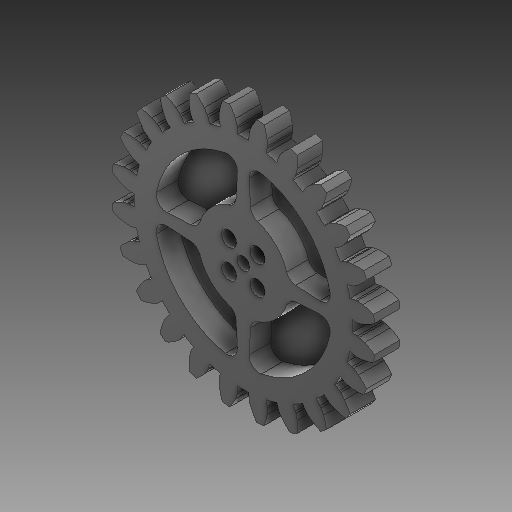
# Autodesk Inventor part: 歯車m2.z24
Saved by Autodesk Inventor 2020 (Build 240168000, 168)
## iProperties
Created: 2019-09-03
Part Number: 歯車m2.z24
Material: アセタール樹脂、黒
Document SubType Name: Modeling
Designer: 雪村
Density: 1.425 g/cm^3
Appearance: 滑らか - 黒
Mass: 8.68564 g
Surface Area: 61.5499 cm^2
Volume: 6.09519 cm^3
Description: ジュラコン 5t
Author: 雪村
Autodesk Inventor part; units mm, degrees
ref_plane "YZ Plane" through (0, 0, 0) normal (1, 0, 0) x (0, 1, 0)
ref_plane "XZ Plane" through (0, 0, 0) normal (0, 1, 0) x (-1, 0, 0)
ref_plane "XY Plane" through (0, 0, 0) normal (0, 0, 1) x (1, 0, 0)
sketch "スケッチ1" plane through (0, 0, 0) normal (0, 0, 1) x (1, 0, 0)
  arc A0 (1.1972, 22.8655) -> (1.1394, 22.5238) centre (3.3501, 22.3258) ccw
  arc A1 (1.5628, 23.9329) -> (1.1972, 22.8655) centre (7.1312, 21.4295) ccw
  arc A2 (2.6831, 25.8612) -> (1.5628, 23.9329) centre (11.2055, 19.6203) ccw
  arc A3 (-4.7616, 22.3962) -> (-4.729, 22.0512) centre (-2.5424, 22.4322) ccw
  arc A4 (-4.6848, 23.5219) -> (-4.7616, 22.3962) centre (1.3418, 22.545) ccw
  arc A5 (-4.1017, 25.6744) -> (-4.6848, 23.5219) centre (5.7456, 21.852) ccw
  arc A6 (-10.3959, 20.4007) -> (-10.2751, 20.0759) centre (-8.2616, 21.0098) ccw
  arc A7 (-10.613, 21.5079) -> (-10.3959, 20.4007) centre (-4.539, 22.1241) ccw
  arc A8 (-10.607, 23.738) -> (-10.613, 21.5079) centre (-0.1059, 22.5945) ccw
  arc A9 (-15.3218, 17.0149) -> (-15.121, 16.7325) centre (-13.4178, 18.1556) ccw
  arc A10 (-15.8181, 18.0282) -> (-15.3218, 17.0149) centre (-10.1104, 20.1955) ccw
  arc A11 (-16.3894, 20.1838) -> (-15.8181, 18.0282) centre (-5.9502, 21.7972) ccw
  arc A12 (-19.2035, 12.4696) -> (-18.9365, 12.2487) centre (-17.6597, 14.0642) ccw
  arc A13 (-19.9451, 13.3199) -> (-19.2035, 12.4696) centre (-14.9929, 16.8905) ccw
  arc A14 (-21.0549, 15.2542) -> (-19.9451, 13.3199) centre (-11.389, 19.5144) ccw
  arc A15 (-21.7765, 7.0744) -> (-21.4614, 6.9302) centre (-20.698, 9.0143) ccw
  arc A16 (-22.713, 7.7038) -> (-21.7765, 7.0744) centre (-18.8536, 12.4346) ccw
  arc A17 (-24.2856, 9.285) -> (-22.713, 7.7038) centre (-16.0516, 15.9018) ccw
  arc A18 (-22.8655, 1.1972) -> (-22.5238, 1.1394) centre (-22.3258, 3.3501) ccw
  arc A19 (-23.9329, 1.5628) -> (-22.8655, 1.1972) centre (-21.4295, 7.1312) ccw
  arc A20 (-25.8612, 2.6831) -> (-23.9329, 1.5628) centre (-19.6203, 11.2055) ccw
  arc A21 (-22.3962, -4.7616) -> (-22.0512, -4.729) centre (-22.4322, -2.5424) ccw
  arc A22 (-23.5219, -4.6848) -> (-22.3962, -4.7616) centre (-22.545, 1.3418) ccw
  arc A23 (-25.6744, -4.1017) -> (-23.5219, -4.6848) centre (-21.852, 5.7456) ccw
  arc A24 (-20.4007, -10.3959) -> (-20.0759, -10.2751) centre (-21.0098, -8.2616) ccw
  arc A25 (-21.5079, -10.613) -> (-20.4007, -10.3959) centre (-22.1241, -4.539) ccw
  arc A26 (-23.738, -10.607) -> (-21.5079, -10.613) centre (-22.5945, -0.1059) ccw
  arc A27 (-17.0149, -15.3218) -> (-16.7325, -15.121) centre (-18.1556, -13.4178) ccw
  arc A28 (-18.0282, -15.8181) -> (-17.0149, -15.3218) centre (-20.1955, -10.1104) ccw
  arc A29 (-20.1838, -16.3894) -> (-18.0282, -15.8181) centre (-21.7972, -5.9502) ccw
  arc A30 (-12.4696, -19.2035) -> (-12.2487, -18.9365) centre (-14.0642, -17.6597) ccw
  arc A31 (-13.3199, -19.9451) -> (-12.4696, -19.2035) centre (-16.8905, -14.9929) ccw
  arc A32 (-15.2542, -21.0549) -> (-13.3199, -19.9451) centre (-19.5144, -11.389) ccw
  arc A33 (-7.0744, -21.7765) -> (-6.9302, -21.4614) centre (-9.0143, -20.698) ccw
  arc A34 (-7.7038, -22.713) -> (-7.0744, -21.7765) centre (-12.4346, -18.8536) ccw
  arc A35 (-9.285, -24.2856) -> (-7.7038, -22.713) centre (-15.9018, -16.0516) ccw
  arc A36 (-1.1972, -22.8655) -> (-1.1394, -22.5238) centre (-3.3501, -22.3258) ccw
  arc A37 (-1.5628, -23.9329) -> (-1.1972, -22.8655) centre (-7.1312, -21.4295) ccw
  arc A38 (-2.6831, -25.8612) -> (-1.5628, -23.9329) centre (-11.2055, -19.6203) ccw
  arc A39 (4.7616, -22.3962) -> (4.729, -22.0512) centre (2.5424, -22.4322) ccw
  arc A40 (4.6848, -23.5219) -> (4.7616, -22.3962) centre (-1.3418, -22.545) ccw
  arc A41 (4.1017, -25.6744) -> (4.6848, -23.5219) centre (-5.7456, -21.852) ccw
  arc A42 (10.3959, -20.4007) -> (10.2751, -20.0759) centre (8.2616, -21.0098) ccw
  arc A43 (10.613, -21.5079) -> (10.3959, -20.4007) centre (4.539, -22.1241) ccw
  arc A44 (10.607, -23.738) -> (10.613, -21.5079) centre (0.1059, -22.5945) ccw
  arc A45 (15.3218, -17.0149) -> (15.121, -16.7325) centre (13.4178, -18.1556) ccw
  arc A46 (15.8181, -18.0282) -> (15.3218, -17.0149) centre (10.1104, -20.1955) ccw
  arc A47 (16.3894, -20.1838) -> (15.8181, -18.0282) centre (5.9502, -21.7972) ccw
  arc A48 (19.2035, -12.4696) -> (18.9365, -12.2487) centre (17.6597, -14.0642) ccw
  arc A49 (19.9451, -13.3199) -> (19.2035, -12.4696) centre (14.9929, -16.8905) ccw
  arc A50 (21.0549, -15.2542) -> (19.9451, -13.3199) centre (11.389, -19.5144) ccw
  arc A51 (21.7765, -7.0744) -> (21.4614, -6.9302) centre (20.698, -9.0143) ccw
  arc A52 (22.713, -7.7038) -> (21.7765, -7.0744) centre (18.8536, -12.4346) ccw
  arc A53 (24.2856, -9.285) -> (22.713, -7.7038) centre (16.0516, -15.9018) ccw
  arc A54 (22.8655, -1.1972) -> (22.5238, -1.1394) centre (22.3258, -3.3501) ccw
  arc A55 (23.9329, -1.5628) -> (22.8655, -1.1972) centre (21.4295, -7.1312) ccw
  arc A56 (25.8612, -2.6831) -> (23.9329, -1.5628) centre (19.6203, -11.2055) ccw
  arc A57 (22.3962, 4.7616) -> (22.0512, 4.729) centre (22.4322, 2.5424) ccw
  arc A58 (23.5219, 4.6848) -> (22.3962, 4.7616) centre (22.545, -1.3418) ccw
  arc A59 (25.6744, 4.1017) -> (23.5219, 4.6848) centre (21.852, -5.7456) ccw
  arc A60 (20.4007, 10.3959) -> (20.0759, 10.2751) centre (21.0098, 8.2616) ccw
  arc A61 (21.5079, 10.613) -> (20.4007, 10.3959) centre (22.1241, 4.539) ccw
  arc A62 (23.738, 10.607) -> (21.5079, 10.613) centre (22.5945, 0.1059) ccw
  arc A63 (17.0149, 15.3218) -> (16.7325, 15.121) centre (18.1556, 13.4178) ccw
  arc A64 (18.0282, 15.8181) -> (17.0149, 15.3218) centre (20.1955, 10.1104) ccw
  arc A65 (20.1838, 16.3894) -> (18.0282, 15.8181) centre (21.7972, 5.9502) ccw
  arc A66 (12.4696, 19.2035) -> (12.2487, 18.9365) centre (14.0642, 17.6597) ccw
  arc A67 (13.3199, 19.9451) -> (12.4696, 19.2035) centre (16.8905, 14.9929) ccw
  arc A68 (15.2542, 21.0549) -> (13.3199, 19.9451) centre (19.5144, 11.389) ccw
  arc A69 (7.0744, 21.7765) -> (6.9302, 21.4614) centre (9.0143, 20.698) ccw
  arc A70 (7.7038, 22.713) -> (7.0744, 21.7765) centre (12.4346, 18.8536) ccw
  arc A71 (9.285, 24.2856) -> (7.7038, 22.713) centre (15.9018, 16.0516) ccw
  arc A72 (-1.1394, 22.5238) -> (-1.1972, 22.8655) centre (-3.3501, 22.3258) ccw
  arc A73 (-1.1972, 22.8655) -> (-1.5628, 23.9329) centre (-7.1312, 21.4295) ccw
  arc A74 (-1.5628, 23.9329) -> (-2.6831, 25.8612) centre (-11.2055, 19.6203) ccw
  arc A75 (-6.9302, 21.4614) -> (-7.0744, 21.7765) centre (-9.0143, 20.698) ccw
  arc A76 (-7.0744, 21.7765) -> (-7.7038, 22.713) centre (-12.4346, 18.8536) ccw
  arc A77 (-7.7038, 22.713) -> (-9.285, 24.2856) centre (-15.9018, 16.0516) ccw
  arc A78 (-12.2487, 18.9365) -> (-12.4696, 19.2035) centre (-14.0642, 17.6597) ccw
  arc A79 (-12.4696, 19.2035) -> (-13.3199, 19.9451) centre (-16.8905, 14.9929) ccw
  arc A80 (-13.3199, 19.9451) -> (-15.2542, 21.0549) centre (-19.5144, 11.389) ccw
  arc A81 (-16.7325, 15.121) -> (-17.0149, 15.3218) centre (-18.1556, 13.4178) ccw
  arc A82 (-17.0149, 15.3218) -> (-18.0282, 15.8181) centre (-20.1955, 10.1104) ccw
  arc A83 (-18.0282, 15.8181) -> (-20.1838, 16.3894) centre (-21.7972, 5.9502) ccw
  arc A84 (-20.0759, 10.2751) -> (-20.4007, 10.3959) centre (-21.0098, 8.2616) ccw
  arc A85 (-20.4007, 10.3959) -> (-21.5079, 10.613) centre (-22.1241, 4.539) ccw
  arc A86 (-21.5079, 10.613) -> (-23.738, 10.607) centre (-22.5945, 0.1059) ccw
  arc A87 (-22.0512, 4.729) -> (-22.3962, 4.7616) centre (-22.4322, 2.5424) ccw
  arc A88 (-22.3962, 4.7616) -> (-23.5219, 4.6848) centre (-22.545, -1.3418) ccw
  arc A89 (-23.5219, 4.6848) -> (-25.6744, 4.1017) centre (-21.852, -5.7456) ccw
  arc A90 (-22.5238, -1.1394) -> (-22.8655, -1.1972) centre (-22.3258, -3.3501) ccw
  arc A91 (-22.8655, -1.1972) -> (-23.9329, -1.5628) centre (-21.4295, -7.1312) ccw
  arc A92 (-23.9329, -1.5628) -> (-25.8612, -2.6831) centre (-19.6203, -11.2055) ccw
  arc A93 (-21.4614, -6.9302) -> (-21.7765, -7.0744) centre (-20.698, -9.0143) ccw
  arc A94 (-21.7765, -7.0744) -> (-22.713, -7.7038) centre (-18.8536, -12.4346) ccw
  arc A95 (-22.713, -7.7038) -> (-24.2856, -9.285) centre (-16.0516, -15.9018) ccw
  arc A96 (-18.9365, -12.2487) -> (-19.2035, -12.4696) centre (-17.6597, -14.0642) ccw
  arc A97 (-19.2035, -12.4696) -> (-19.9451, -13.3199) centre (-14.9929, -16.8905) ccw
  arc A98 (-19.9451, -13.3199) -> (-21.0549, -15.2542) centre (-11.389, -19.5144) ccw
  arc A99 (-15.121, -16.7325) -> (-15.3218, -17.0149) centre (-13.4178, -18.1556) ccw
  arc A100 (-15.3218, -17.0149) -> (-15.8181, -18.0282) centre (-10.1104, -20.1955) ccw
  arc A101 (-15.8181, -18.0282) -> (-16.3894, -20.1838) centre (-5.9502, -21.7972) ccw
  arc A102 (-10.2751, -20.0759) -> (-10.3959, -20.4007) centre (-8.2616, -21.0098) ccw
  arc A103 (-10.3959, -20.4007) -> (-10.613, -21.5079) centre (-4.539, -22.1241) ccw
  arc A104 (-10.613, -21.5079) -> (-10.607, -23.738) centre (-0.1059, -22.5945) ccw
  arc A105 (-4.729, -22.0512) -> (-4.7616, -22.3962) centre (-2.5424, -22.4322) ccw
  arc A106 (-4.7616, -22.3962) -> (-4.6848, -23.5219) centre (1.3418, -22.545) ccw
  arc A107 (-4.6848, -23.5219) -> (-4.1017, -25.6744) centre (5.7456, -21.852) ccw
  arc A108 (1.1394, -22.5238) -> (1.1972, -22.8655) centre (3.3501, -22.3258) ccw
  arc A109 (1.1972, -22.8655) -> (1.5628, -23.9329) centre (7.1312, -21.4295) ccw
  arc A110 (1.5628, -23.9329) -> (2.6831, -25.8612) centre (11.2055, -19.6203) ccw
  arc A111 (6.9302, -21.4614) -> (7.0744, -21.7765) centre (9.0143, -20.698) ccw
  arc A112 (7.0744, -21.7765) -> (7.7038, -22.713) centre (12.4346, -18.8536) ccw
  arc A113 (7.7038, -22.713) -> (9.285, -24.2856) centre (15.9018, -16.0516) ccw
  arc A114 (12.2487, -18.9365) -> (12.4696, -19.2035) centre (14.0642, -17.6597) ccw
  arc A115 (12.4696, -19.2035) -> (13.3199, -19.9451) centre (16.8905, -14.9929) ccw
  arc A116 (13.3199, -19.9451) -> (15.2542, -21.0549) centre (19.5144, -11.389) ccw
  arc A117 (16.7325, -15.121) -> (17.0149, -15.3218) centre (18.1556, -13.4178) ccw
  arc A118 (17.0149, -15.3218) -> (18.0282, -15.8181) centre (20.1955, -10.1104) ccw
  arc A119 (18.0282, -15.8181) -> (20.1838, -16.3894) centre (21.7972, -5.9502) ccw
  arc A120 (20.0759, -10.2751) -> (20.4007, -10.3959) centre (21.0098, -8.2616) ccw
  arc A121 (20.4007, -10.3959) -> (21.5079, -10.613) centre (22.1241, -4.539) ccw
  arc A122 (21.5079, -10.613) -> (23.738, -10.607) centre (22.5945, -0.1059) ccw
  arc A123 (22.0512, -4.729) -> (22.3962, -4.7616) centre (22.4322, -2.5424) ccw
  arc A124 (22.3962, -4.7616) -> (23.5219, -4.6848) centre (22.545, 1.3418) ccw
  arc A125 (23.5219, -4.6848) -> (25.6744, -4.1017) centre (21.852, 5.7456) ccw
  arc A126 (22.5238, 1.1394) -> (22.8655, 1.1972) centre (22.3258, 3.3501) ccw
  arc A127 (22.8655, 1.1972) -> (23.9329, 1.5628) centre (21.4295, 7.1312) ccw
  arc A128 (23.9329, 1.5628) -> (25.8612, 2.6831) centre (19.6203, 11.2055) ccw
  arc A129 (21.4614, 6.9302) -> (21.7765, 7.0744) centre (20.698, 9.0143) ccw
  arc A130 (21.7765, 7.0744) -> (22.713, 7.7038) centre (18.8536, 12.4346) ccw
  arc A131 (22.713, 7.7038) -> (24.2856, 9.285) centre (16.0516, 15.9018) ccw
  arc A132 (18.9365, 12.2487) -> (19.2035, 12.4696) centre (17.6597, 14.0642) ccw
  arc A133 (19.2035, 12.4696) -> (19.9451, 13.3199) centre (14.9929, 16.8905) ccw
  arc A134 (19.9451, 13.3199) -> (21.0549, 15.2542) centre (11.389, 19.5144) ccw
  arc A135 (15.121, 16.7325) -> (15.3218, 17.0149) centre (13.4178, 18.1556) ccw
  arc A136 (15.3218, 17.0149) -> (15.8181, 18.0282) centre (10.1104, 20.1955) ccw
  arc A137 (15.8181, 18.0282) -> (16.3894, 20.1838) centre (5.9502, 21.7972) ccw
  arc A138 (10.2751, 20.0759) -> (10.3959, 20.4007) centre (8.2616, 21.0098) ccw
  arc A139 (10.3959, 20.4007) -> (10.613, 21.5079) centre (4.539, 22.1241) ccw
  arc A140 (10.613, 21.5079) -> (10.607, 23.738) centre (0.1059, 22.5945) ccw
  arc A141 (4.729, 22.0512) -> (4.7616, 22.3962) centre (2.5424, 22.4322) ccw
  arc A142 (4.7616, 22.3962) -> (4.6848, 23.5219) centre (-1.3418, 22.545) ccw
  arc A143 (4.6848, 23.5219) -> (4.1017, 25.6744) centre (-5.7456, 21.852) ccw
  arc A144 (1.0863, 21.4725) -> (-1.0863, 21.4725) centre (0, 0) ccw
  arc A145 (-4.5083, 21.022) -> (-6.6068, 20.4597) centre (0, 0) ccw
  arc A146 (-9.7955, 19.1389) -> (-11.677, 18.0526) centre (0, 0) ccw
  arc A147 (-14.4153, 15.9515) -> (-15.9515, 14.4153) centre (0, 0) ccw
  arc A148 (-18.0526, 11.677) -> (-19.1389, 9.7955) centre (0, 0) ccw
  arc A149 (-20.4597, 6.6068) -> (-21.022, 4.5083) centre (0, 0) ccw
  arc A150 (-21.4725, 1.0863) -> (-21.4725, -1.0863) centre (0, 0) ccw
  arc A151 (-21.022, -4.5083) -> (-20.4597, -6.6068) centre (0, 0) ccw
  arc A152 (-19.1389, -9.7955) -> (-18.0526, -11.677) centre (0, 0) ccw
  arc A153 (-15.9515, -14.4153) -> (-14.4153, -15.9515) centre (0, 0) ccw
  arc A154 (-11.677, -18.0526) -> (-9.7955, -19.1389) centre (0, 0) ccw
  arc A155 (-6.6068, -20.4597) -> (-4.5083, -21.022) centre (0, 0) ccw
  arc A156 (-1.0863, -21.4725) -> (1.0863, -21.4725) centre (0, 0) ccw
  arc A157 (4.5083, -21.022) -> (6.6068, -20.4597) centre (0, 0) ccw
  arc A158 (9.7955, -19.1389) -> (11.677, -18.0526) centre (0, 0) ccw
  arc A159 (14.4153, -15.9515) -> (15.9515, -14.4153) centre (0, 0) ccw
  arc A160 (18.0526, -11.677) -> (19.1389, -9.7955) centre (0, 0) ccw
  arc A161 (20.4597, -6.6068) -> (21.022, -4.5083) centre (0, 0) ccw
  arc A162 (21.4725, -1.0863) -> (21.4725, 1.0863) centre (0, 0) ccw
  arc A163 (21.022, 4.5083) -> (20.4597, 6.6068) centre (0, 0) ccw
  arc A164 (19.1389, 9.7955) -> (18.0526, 11.677) centre (0, 0) ccw
  arc A165 (15.9515, 14.4153) -> (14.4153, 15.9515) centre (0, 0) ccw
  arc A166 (11.677, 18.0526) -> (9.7955, 19.1389) centre (0, 0) ccw
  arc A167 (6.6068, 20.4597) -> (4.5083, 21.022) centre (0, 0) ccw
  arc A168 (-2.6831, 25.8612) -> (-4.1017, 25.6744) centre (0, 0) ccw
  arc A169 (-9.285, 24.2856) -> (-10.607, 23.738) centre (0, 0) ccw
  arc A170 (-15.2542, 21.0549) -> (-16.3894, 20.1838) centre (0, 0) ccw
  arc A171 (-20.1838, 16.3894) -> (-21.0549, 15.2542) centre (0, 0) ccw
  arc A172 (-23.738, 10.607) -> (-24.2856, 9.285) centre (0, 0) ccw
  arc A173 (-25.6744, 4.1017) -> (-25.8612, 2.6831) centre (0, 0) ccw
  arc A174 (-25.8612, -2.6831) -> (-25.6744, -4.1017) centre (0, 0) ccw
  arc A175 (-24.2856, -9.285) -> (-23.738, -10.607) centre (0, 0) ccw
  arc A176 (-21.0549, -15.2542) -> (-20.1838, -16.3894) centre (0, 0) ccw
  arc A177 (-16.3894, -20.1838) -> (-15.2542, -21.0549) centre (0, 0) ccw
  arc A178 (-10.607, -23.738) -> (-9.285, -24.2856) centre (0, 0) ccw
  arc A179 (-4.1017, -25.6744) -> (-2.6831, -25.8612) centre (0, 0) ccw
  arc A180 (2.6831, -25.8612) -> (4.1017, -25.6744) centre (0, 0) ccw
  arc A181 (9.285, -24.2856) -> (10.607, -23.738) centre (0, 0) ccw
  arc A182 (15.2542, -21.0549) -> (16.3894, -20.1838) centre (0, 0) ccw
  arc A183 (20.1838, -16.3894) -> (21.0549, -15.2542) centre (0, 0) ccw
  arc A184 (23.738, -10.607) -> (24.2856, -9.285) centre (0, 0) ccw
  arc A185 (25.6744, -4.1017) -> (25.8612, -2.6831) centre (0, 0) ccw
  arc A186 (25.8612, 2.6831) -> (25.6744, 4.1017) centre (0, 0) ccw
  arc A187 (24.2856, 9.285) -> (23.738, 10.607) centre (0, 0) ccw
  arc A188 (21.0549, 15.2542) -> (20.1838, 16.3894) centre (0, 0) ccw
  arc A189 (16.3894, 20.1838) -> (15.2542, 21.0549) centre (0, 0) ccw
  arc A190 (10.607, 23.738) -> (9.285, 24.2856) centre (0, 0) ccw
  arc A191 (4.1017, 25.6744) -> (2.6831, 25.8612) centre (0, 0) ccw
  line L0 (1.0863, 21.4725) -> (1.1394, 22.5238)
  line L1 (-4.5083, 21.022) -> (-4.729, 22.0512)
  line L2 (-9.7955, 19.1389) -> (-10.2751, 20.0759)
  line L3 (-14.4153, 15.9515) -> (-15.121, 16.7325)
  line L4 (-18.0526, 11.677) -> (-18.9365, 12.2487)
  line L5 (-20.4597, 6.6068) -> (-21.4614, 6.9302)
  line L6 (-21.4725, 1.0863) -> (-22.5238, 1.1394)
  line L7 (-21.022, -4.5083) -> (-22.0512, -4.729)
  line L8 (-19.1389, -9.7955) -> (-20.0759, -10.2751)
  line L9 (-15.9515, -14.4153) -> (-16.7325, -15.121)
  line L10 (-11.677, -18.0526) -> (-12.2487, -18.9365)
  line L11 (-6.6068, -20.4597) -> (-6.9302, -21.4614)
  line L12 (-1.0863, -21.4725) -> (-1.1394, -22.5238)
  line L13 (4.5083, -21.022) -> (4.729, -22.0512)
  line L14 (9.7955, -19.1389) -> (10.2751, -20.0759)
  line L15 (14.4153, -15.9515) -> (15.121, -16.7325)
  line L16 (18.0526, -11.677) -> (18.9365, -12.2487)
  line L17 (20.4597, -6.6068) -> (21.4614, -6.9302)
  line L18 (21.4725, -1.0863) -> (22.5238, -1.1394)
  line L19 (21.022, 4.5083) -> (22.0512, 4.729)
  line L20 (19.1389, 9.7955) -> (20.0759, 10.2751)
  line L21 (15.9515, 14.4153) -> (16.7325, 15.121)
  line L22 (11.677, 18.0526) -> (12.2487, 18.9365)
  line L23 (6.6068, 20.4597) -> (6.9302, 21.4614)
  line L24 (-1.0863, 21.4725) -> (-1.1394, 22.5238)
  line L25 (-6.6068, 20.4597) -> (-6.9302, 21.4614)
  line L26 (-11.677, 18.0526) -> (-12.2487, 18.9365)
  line L27 (-15.9515, 14.4153) -> (-16.7325, 15.121)
  line L28 (-19.1389, 9.7955) -> (-20.0759, 10.2751)
  line L29 (-21.022, 4.5083) -> (-22.0512, 4.729)
  line L30 (-21.4725, -1.0863) -> (-22.5238, -1.1394)
  line L31 (-20.4597, -6.6068) -> (-21.4614, -6.9302)
  line L32 (-18.0526, -11.677) -> (-18.9365, -12.2487)
  line L33 (-14.4153, -15.9515) -> (-15.121, -16.7325)
  line L34 (-9.7955, -19.1389) -> (-10.2751, -20.0759)
  line L35 (-4.5083, -21.022) -> (-4.729, -22.0512)
  line L36 (1.0863, -21.4725) -> (1.1394, -22.5238)
  line L37 (6.6068, -20.4597) -> (6.9302, -21.4614)
  line L38 (11.677, -18.0526) -> (12.2487, -18.9365)
  line L39 (15.9515, -14.4153) -> (16.7325, -15.121)
  line L40 (19.1389, -9.7955) -> (20.0759, -10.2751)
  line L41 (21.022, -4.5083) -> (22.0512, -4.729)
  line L42 (21.4725, 1.0863) -> (22.5238, 1.1394)
  line L43 (20.4597, 6.6068) -> (21.4614, 6.9302)
  line L44 (18.0526, 11.677) -> (18.9365, 12.2487)
  line L45 (14.4153, 15.9515) -> (15.121, 16.7325)
  line L46 (9.7955, 19.1389) -> (10.2751, 20.0759)
  line L47 (4.5083, 21.022) -> (4.729, 22.0512)
  line L48 (-28, 0) -> (28, 0)
  line L49 (0, -28) -> (0, 28)
  line L50 (46, 26) -> (116, 26)
  line L51 (46, 18) -> (116, 18)
  line L52 (46, 10) -> (116, 10)
  line L53 (46, 2) -> (116, 2)
  line L54 (46, -6) -> (116, -6)
  line L55 (46, -14) -> (116, -14)
  line L56 (46, -22) -> (116, -22)
  line L57 (46, -30) -> (116, -30)
  line L58 (46, -38) -> (116, -38)
  line L59 (46, -46) -> (116, -46)
  line L60 (46, -54) -> (116, -54)
  line L61 (46, -62) -> (116, -62)
  line L62 (46, -70) -> (116, -70)
  line L63 (46, 26) -> (46, -70)
  line L64 (116, 26) -> (116, -70)
  line L65 (81, 18) -> (81, -70)
  point P0 (0, 0)
  point P1 (52, 20)
  point P2 (54.5, 12)
  point P3 (54.5, 4)
  point P4 (52, -4)
  point P5 (54.5, -12)
  point P6 (49.5, -20)
  point P7 (52, -28)
  point P8 (52, -36)
  point P9 (52, -44)
  point P10 (54.5, -52)
  point P11 (54.5, -60)
  point P12 (52, -68)
  point P13 (82, 12)
  point P14 (97, 4)
  point P15 (98.25, -4)
  point P16 (94.5, -12)
  point P17 (97, -20)
  point P18 (90.75, -28)
  point P19 (97, -36)
  point P20 (97, -44)
  point P21 (92, -52)
  point P22 (1, 41.5)
  point P23 (1, 35.5)
  point P24 (17.1875, 41.5)
  point P25 (19.3125, 35.5)
  constraints: 288 point on circle, 144 centre point, 128 end point, 14 horizontal, 2 horizontal alignment, 2 midpoint, 2 vertical, 2 vertical alignment, 827 other
extrude "押し出し1" add sketch "スケッチ1" along normal blind 5 contours A1 A2 A191 A143 A142 A141 L47 A167 L23 A69 A70 A71 A190 A140 A139 A138 L46 A166 L22 A66 A67 A68 A189 A137 A136 A135 L45 A165 L21 A63 A64 A65 A188 A134 A133 A132 L44 A164 L20 A60 A61 A62 A187 A131 A130 A129 L43 A163 L19 A57 A58 A59 A186 A128 A127 A126 L42 A162 L48 L49 A144 L0 A0 | L49 L48 A150 L6 A18 A19 A20 A173 A89 A88 A87 L29 A149 L5 A15 A16 A17 A172 A86 A85 A84 L28 A148 L4 A12 A13 A14 A171 A83 A82 A81 L27 A147 L3 A9 A10 A11 A170 A80 A79 A78 L26 A146 L2 A6 A7 A8 A169 A77 A76 A75 L25 A145 L1 A3 A4 A5 A168 A74 A73 A72 L24 A144 | L49 A156 L12 A36 A37 A38 A179 A107 A106 A105 L35 A155 L11 A33 A34 A35 A178 A104 A103 A102 L34 A154 L10 A30 A31 A32 A177 A101 A100 A99 L33 A153 L9 A27 A28 A29 A176 A98 A97 A96 L32 A152 L8 A24 A25 A26 A175 A95 A94 A93 L31 A151 L7 A21 A22 A23 A174 A92 A91 A90 L30 A150 L48 | L48 A162 L18 A54 A55 A56 A185 A125 A124 A123 L41 A161 L17 A51 A52 A53 A184 A122 A121 A120 L40 A160 L16 A48 A49 A50 A183 A119 A118 A117 L39 A159 L15 A45 A46 A47 A182 A116 A115 A114 L38 A158 L14 A42 A43 A44 A181 A113 A112 A111 L37 A157 L13 A39 A40 A41 A180 A110 A109 A108 L36 A156 L49
sketch "スケッチ2" plane through (0, 0, 5) normal (0, 0, 1) x (1, 0, 0)
  line L0 (-2.8, 2.8) -> (2.8, 2.8) construction
  line L1 (2.8, 2.8) -> (2.8, -2.8) construction
  line L2 (2.8, -2.8) -> (-2.8, -2.8) construction
  line L3 (-2.8, -2.8) -> (-2.8, 2.8) construction
  circle A0 centre (-2.8, 2.8) radius 1.5
  circle A1 centre (2.8, 2.8) radius 1.5
  circle A2 centre (2.8, -2.8) radius 1.5
  circle A3 centre (-2.8, -2.8) radius 1.5
  point P0 (0, 0)
  point P1 (0, 0)
  dimension "d2" = 3
  dimension "d3" = 3
  dimension "d4" = 3
  dimension "d5" = 3
  dimension "d6" = 5.6
  constraints: 8 end point, 5 coincident, 4 centre point, 1 horizontal, 9 other
  measures "d2" diameter of A0
  measures "d3" diameter of A1
  measures "d4" diameter of A2
  measures "d5" diameter of A3
  measures "d6" distance of L0.start L0.end
extrude "押し出し2" cut sketch "スケッチ2" against normal through all
sketch "スケッチ3" plane through (0, 0, 5) normal (0, 0, 1) x (1, 0, 0)
  circle A0 centre (0, 0) radius 1.25
  dimension "d9" = 2.5
  constraints: 1 centre point, 1 coincident
  measures "d9" diameter of A0
extrude "押し出し3" cut sketch "スケッチ3" against normal through all
sketch "スケッチ4" plane through (0, 0, 0) normal (0, 0, -1) x (-1, 0, 0)
  circle A0 centre (0, 0) radius 9
  circle A1 centre (0, 0) radius 6
  circle A2 centre (0, 0) radius 17.5
  line L0 (0, 15.6403) -> (0, -15.6403)
  line L1 (-15.4429, 0) -> (15.4429, 0)
  line L2 (-1, 17.4714) -> (-1.5, 8.8741)
  line L3 (1, 17.4714) -> (1.5, 8.8741)
  line L4 (8.8741, 1.5) -> (17.4714, 1)
  line L5 (8.8741, -1.5) -> (17.4714, -1)
  circle A3 centre (0, 0) radius 9
  line L6 (1.5, -8.8741) -> (1, -17.4714)
  line L7 (-17.4714, 1) -> (-8.8741, 1.5)
  line L8 (-17.4714, -1) -> (-8.8741, -1.5)
  line L9 (-1.5, -8.8741) -> (-1, -17.4714)
  circle A4 centre (0, 0) radius 6
  circle A5 centre (0, 0) radius 21.5
  circle A6 centre (0, 0) radius 6
  circle A7 centre (0, 0) radius 1.25 projected
  point P0 (16.9761, 62.7038)
  point P1 (20.9761, 62.7038)
  point P2 (11.2302, 68.4498)
  point P3 (11.2302, 72.4498)
  point P4 (16.9761, 62.7038)
  point P5 (20.9761, 62.7038)
  point P6 (11.2302, 68.4498)
  point P7 (11.2302, 72.4498)
  point P8 (-9.7955, 19.1389)
  point P9 (-2, -7.746)
  point P10 (2, -7.746)
  point P11 (-7.746, -2)
  point P12 (-7.746, 2)
  point P13 (-9.7955, 19.1389)
  point P14 (-1.5, -7.8581)
  point P15 (-7.8581, -1.5)
  point P16 (1.5, -7.8581)
  point P17 (-7.8581, 1.5)
  point P18 (-9.7955, 19.1389)
  dimension "d28" = 4
  dimension "d12" = 1
  dimension "d13" = 1
  dimension "d14" = 1
  dimension "d15" = 1
  dimension "d16" = 1
  dimension "d17" = 1
  dimension "d18" = 1
  dimension "d19" = 1
  dimension "d20" = 1.5
  dimension "d21" = 1.5
  dimension "d22" = 1.5
  dimension "d23" = 1.5
  dimension "d24" = 1.5
  dimension "d25" = 1.5
  dimension "d26" = 1.5
  dimension "d27" = 1.5
  dimension "d29" = 3
  dimension "d30" = 12
  constraints: 20 end point, 5 concentric, 4 centre point, 4 coincident, 4 point on circle, 2 midpoint, 1 horizontal, 1 vertical, 23 other
  measures "d12" distance from line of L0 L2.start
  measures "d13" distance from line of L3.start L0
  measures "d14" distance from line of L1 L4.end
  measures "d15" distance from line of L5.end L1
  measures "d16" distance from line of L0 L6.end
  measures "d17" distance from line of L0 L9.end
  measures "d18" distance from line of L1 L8.start
  measures "d19" distance from line of L1 L7.start
  measures "d20" distance from line of L0 L2.end
  measures "d21" distance from line of L0 L3.end
  measures "d22" distance from line of L1 L4.start
  measures "d23" distance from line of L5.start L1
  measures "d24" distance from line of L0 L6.start
  measures "d25" distance from line of L9.start L0
  measures "d26" distance from line of L1 L8.end
  measures "d27" distance from line of L1 L7.end
  measures "d29" radial gap between concentric circles of A0 A1
  measures "d30" diameter of A1
extrude "押し出し4" cut sketch "スケッチ4" against normal through all contours A0 L3 A2 L4 | L5 A2 L6 A0 | A0 L7 A2 L2 | L9 A2 L8 A0
fillet "フィレット1" radius 2 16 edges at (17.4714, -1, 2.5) (17.4714, 1, 2.5) (8.8741, -1.5, 2.5) (8.8741, 1.5, 2.5) (1.5, 8.8741, 2.5) (-1.5, 8.8741, 2.5) (1, 17.4714, 2.5) (-1, 17.4714, 2.5) (-17.4714, 1, 2.5) (-17.4714, -1, 2.5) (-8.8741, 1.5, 2.5) (-8.8741, -1.5, 2.5) (1.5, -8.8741, 2.5) (-1.5, -8.8741, 2.5) (1, -17.4714, 2.5) (-1, -17.4714, 2.5)
sketch "スケッチ5" plane through (0, 0, 0) normal (0, 0, -1) x (-1, 0, 0)
  arc A0 (-8.5563, -2.791) -> (-2.791, -8.5563) centre (0, 0) ccw projected
  arc A1 (-1.4147, -10.3416) -> (-2.791, -8.5563) centre (-3.4113, -10.4577) ccw projected
  line L0 (-1.4147, -10.3416) -> (-1.1401, -15.0632) projected
  arc A2 (-3.5414, -17.1379) -> (-1.1401, -15.0632) centre (-3.1367, -15.1793) ccw projected
  arc A3 (-17.1379, -3.5414) -> (-3.5414, -17.1379) centre (0, 0) ccw projected
  arc A4 (-15.0632, -1.1401) -> (-17.1379, -3.5414) centre (-15.1793, -3.1367) ccw projected
  line L1 (-15.0632, -1.1401) -> (-10.3416, -1.4147) projected
  arc A5 (-8.5563, -2.791) -> (-10.3416, -1.4147) centre (-10.4577, -3.4113) ccw projected
  line L2 (-1.1401, 15.0632) -> (-1.4147, 10.3416) projected
  arc A6 (-2.791, 8.5563) -> (-1.4147, 10.3416) centre (-3.4113, 10.4577) ccw projected
  arc A7 (-2.791, 8.5563) -> (-8.5563, 2.791) centre (0, 0) ccw projected
  arc A8 (-10.3416, 1.4147) -> (-8.5563, 2.791) centre (-10.4577, 3.4113) ccw projected
  line L3 (-10.3416, 1.4147) -> (-15.0632, 1.1401) projected
  arc A9 (-17.1379, 3.5414) -> (-15.0632, 1.1401) centre (-15.1793, 3.1367) ccw projected
  arc A10 (-3.5414, 17.1379) -> (-17.1379, 3.5414) centre (0, 0) ccw projected
  arc A11 (-1.1401, 15.0632) -> (-3.5414, 17.1379) centre (-3.1367, 15.1793) ccw projected
  arc A12 (3.5414, -17.1379) -> (17.1379, -3.5414) centre (0, 0) ccw projected
  arc A13 (1.1401, -15.0632) -> (3.5414, -17.1379) centre (3.1367, -15.1793) ccw projected
  line L4 (1.1401, -15.0632) -> (1.4147, -10.3416) projected
  arc A14 (2.791, -8.5563) -> (1.4147, -10.3416) centre (3.4113, -10.4577) ccw projected
  arc A15 (2.791, -8.5563) -> (8.5563, -2.791) centre (0, 0) ccw projected
  arc A16 (10.3416, -1.4147) -> (8.5563, -2.791) centre (10.4577, -3.4113) ccw projected
  line L5 (10.3416, -1.4147) -> (15.0632, -1.1401) projected
  arc A17 (17.1379, -3.5414) -> (15.0632, -1.1401) centre (15.1793, -3.1367) ccw projected
  arc A18 (17.1379, 3.5414) -> (3.5414, 17.1379) centre (0, 0) ccw projected
  arc A19 (15.0632, 1.1401) -> (17.1379, 3.5414) centre (15.1793, 3.1367) ccw projected
  line L6 (15.0632, 1.1401) -> (10.3416, 1.4147) projected
  arc A20 (8.5563, 2.791) -> (10.3416, 1.4147) centre (10.4577, 3.4113) ccw projected
  arc A21 (8.5563, 2.791) -> (2.791, 8.5563) centre (0, 0) ccw projected
  arc A22 (1.4147, 10.3416) -> (2.791, 8.5563) centre (3.4113, 10.4577) ccw projected
  line L7 (1.4147, 10.3416) -> (1.1401, 15.0632) projected
  arc A23 (3.5414, 17.1379) -> (1.1401, 15.0632) centre (3.1367, 15.1793) ccw projected
  circle A24 centre (0, 0) radius 1.25 projected
  circle A25 centre (-2.8, -2.8) radius 1.5 projected
  circle A26 centre (-2.8, 2.8) radius 1.5 projected
  circle A27 centre (2.8, 2.8) radius 1.5 projected
  circle A28 centre (2.8, -2.8) radius 1.5 projected
  arc A29 (-15.8181, -18.0282) -> (-16.3894, -20.1838) centre (-5.9502, -21.7972) ccw projected
  arc A30 (-16.3894, -20.1838) -> (-15.2542, -21.0549) centre (0, 0) ccw projected
  arc A31 (-15.2542, -21.0549) -> (-13.3199, -19.9451) centre (-19.5144, -11.389) ccw projected
  arc A32 (-13.3199, -19.9451) -> (-12.4696, -19.2035) centre (-16.8905, -14.9929) ccw projected
  arc A33 (-12.4696, -19.2035) -> (-12.2487, -18.9365) centre (-14.0642, -17.6597) ccw projected
  line L8 (-11.677, -18.0526) -> (-12.2487, -18.9365) projected
  arc A34 (-11.677, -18.0526) -> (-9.7955, -19.1389) centre (0, 0) ccw projected
  line L9 (-10.2751, -20.0759) -> (-9.7955, -19.1389) projected
  arc A35 (-10.2751, -20.0759) -> (-10.3959, -20.4007) centre (-8.2616, -21.0098) ccw projected
  arc A36 (-10.3959, -20.4007) -> (-10.613, -21.5079) centre (-4.539, -22.1241) ccw projected
  arc A37 (-10.613, -21.5079) -> (-10.607, -23.738) centre (-0.1059, -22.5945) ccw projected
  arc A38 (-10.607, -23.738) -> (-9.285, -24.2856) centre (0, 0) ccw projected
  arc A39 (-9.285, -24.2856) -> (-7.7038, -22.713) centre (-15.9018, -16.0516) ccw projected
  arc A40 (-7.7038, -22.713) -> (-7.0744, -21.7765) centre (-12.4346, -18.8536) ccw projected
  arc A41 (-7.0744, -21.7765) -> (-6.9302, -21.4614) centre (-9.0143, -20.698) ccw projected
  line L10 (-6.6068, -20.4597) -> (-6.9302, -21.4614) projected
  arc A42 (-6.6068, -20.4597) -> (-4.5083, -21.022) centre (0, 0) ccw projected
  line L11 (-4.729, -22.0512) -> (-4.5083, -21.022) projected
  arc A43 (-4.729, -22.0512) -> (-4.7616, -22.3962) centre (-2.5424, -22.4322) ccw projected
  arc A44 (-4.7616, -22.3962) -> (-4.6848, -23.5219) centre (1.3418, -22.545) ccw projected
  arc A45 (-4.6848, -23.5219) -> (-4.1017, -25.6744) centre (5.7456, -21.852) ccw projected
  arc A46 (-4.1017, -25.6744) -> (-2.6831, -25.8612) centre (0, 0) ccw projected
  arc A47 (-2.6831, -25.8612) -> (-1.5628, -23.9329) centre (-11.2055, -19.6203) ccw projected
  arc A48 (-1.5628, -23.9329) -> (-1.1972, -22.8655) centre (-7.1312, -21.4295) ccw projected
  arc A49 (-1.1972, -22.8655) -> (-1.1394, -22.5238) centre (-3.3501, -22.3258) ccw projected
  line L12 (-1.0863, -21.4725) -> (-1.1394, -22.5238) projected
  arc A50 (-1.0863, -21.4725) -> (1.0863, -21.4725) centre (0, 0) ccw projected
  line L13 (1.1394, -22.5238) -> (1.0863, -21.4725) projected
  arc A51 (1.1394, -22.5238) -> (1.1972, -22.8655) centre (3.3501, -22.3258) ccw projected
  arc A52 (1.1972, -22.8655) -> (1.5628, -23.9329) centre (7.1312, -21.4295) ccw projected
  arc A53 (1.5628, -23.9329) -> (2.6831, -25.8612) centre (11.2055, -19.6203) ccw projected
  arc A54 (2.6831, -25.8612) -> (4.1017, -25.6744) centre (0, 0) ccw projected
  arc A55 (4.1017, -25.6744) -> (4.6848, -23.5219) centre (-5.7456, -21.852) ccw projected
  arc A56 (4.6848, -23.5219) -> (4.7616, -22.3962) centre (-1.3418, -22.545) ccw projected
  arc A57 (4.7616, -22.3962) -> (4.729, -22.0512) centre (2.5424, -22.4322) ccw projected
  line L14 (4.5083, -21.022) -> (4.729, -22.0512) projected
  arc A58 (4.5083, -21.022) -> (6.6068, -20.4597) centre (0, 0) ccw projected
  line L15 (6.9302, -21.4614) -> (6.6068, -20.4597) projected
  arc A59 (6.9302, -21.4614) -> (7.0744, -21.7765) centre (9.0143, -20.698) ccw projected
  arc A60 (7.0744, -21.7765) -> (7.7038, -22.713) centre (12.4346, -18.8536) ccw projected
  arc A61 (7.7038, -22.713) -> (9.285, -24.2856) centre (15.9018, -16.0516) ccw projected
  arc A62 (9.285, -24.2856) -> (10.607, -23.738) centre (0, 0) ccw projected
  arc A63 (10.607, -23.738) -> (10.613, -21.5079) centre (0.1059, -22.5945) ccw projected
  arc A64 (10.613, -21.5079) -> (10.3959, -20.4007) centre (4.539, -22.1241) ccw projected
  arc A65 (10.3959, -20.4007) -> (10.2751, -20.0759) centre (8.2616, -21.0098) ccw projected
  line L16 (9.7955, -19.1389) -> (10.2751, -20.0759) projected
  arc A66 (9.7955, -19.1389) -> (11.677, -18.0526) centre (0, 0) ccw projected
  line L17 (12.2487, -18.9365) -> (11.677, -18.0526) projected
  arc A67 (12.2487, -18.9365) -> (12.4696, -19.2035) centre (14.0642, -17.6597) ccw projected
  arc A68 (12.4696, -19.2035) -> (13.3199, -19.9451) centre (16.8905, -14.9929) ccw projected
  arc A69 (13.3199, -19.9451) -> (15.2542, -21.0549) centre (19.5144, -11.389) ccw projected
  arc A70 (15.2542, -21.0549) -> (16.3894, -20.1838) centre (0, 0) ccw projected
  arc A71 (16.3894, -20.1838) -> (15.8181, -18.0282) centre (5.9502, -21.7972) ccw projected
  arc A72 (15.8181, -18.0282) -> (15.3218, -17.0149) centre (10.1104, -20.1955) ccw projected
  arc A73 (15.3218, -17.0149) -> (15.121, -16.7325) centre (13.4178, -18.1556) ccw projected
  line L18 (14.4153, -15.9515) -> (15.121, -16.7325) projected
  arc A74 (14.4153, -15.9515) -> (15.9515, -14.4153) centre (0, 0) ccw projected
  line L19 (16.7325, -15.121) -> (15.9515, -14.4153) projected
  arc A75 (16.7325, -15.121) -> (17.0149, -15.3218) centre (18.1556, -13.4178) ccw projected
  arc A76 (17.0149, -15.3218) -> (18.0282, -15.8181) centre (20.1955, -10.1104) ccw projected
  arc A77 (18.0282, -15.8181) -> (20.1838, -16.3894) centre (21.7972, -5.9502) ccw projected
  arc A78 (20.1838, -16.3894) -> (21.0549, -15.2542) centre (0, 0) ccw projected
  arc A79 (21.0549, -15.2542) -> (19.9451, -13.3199) centre (11.389, -19.5144) ccw projected
  arc A80 (19.9451, -13.3199) -> (19.2035, -12.4696) centre (14.9929, -16.8905) ccw projected
  arc A81 (19.2035, -12.4696) -> (18.9365, -12.2487) centre (17.6597, -14.0642) ccw projected
  line L20 (18.0526, -11.677) -> (18.9365, -12.2487) projected
  arc A82 (18.0526, -11.677) -> (19.1389, -9.7955) centre (0, 0) ccw projected
  line L21 (20.0759, -10.2751) -> (19.1389, -9.7955) projected
  arc A83 (20.0759, -10.2751) -> (20.4007, -10.3959) centre (21.0098, -8.2616) ccw projected
  arc A84 (20.4007, -10.3959) -> (21.5079, -10.613) centre (22.1241, -4.539) ccw projected
  arc A85 (21.5079, -10.613) -> (23.738, -10.607) centre (22.5945, -0.1059) ccw projected
  arc A86 (23.738, -10.607) -> (24.2856, -9.285) centre (0, 0) ccw projected
  arc A87 (24.2856, -9.285) -> (22.713, -7.7038) centre (16.0516, -15.9018) ccw projected
  arc A88 (22.713, -7.7038) -> (21.7765, -7.0744) centre (18.8536, -12.4346) ccw projected
  arc A89 (21.7765, -7.0744) -> (21.4614, -6.9302) centre (20.698, -9.0143) ccw projected
  line L22 (20.4597, -6.6068) -> (21.4614, -6.9302) projected
  arc A90 (20.4597, -6.6068) -> (21.022, -4.5083) centre (0, 0) ccw projected
  line L23 (22.0512, -4.729) -> (21.022, -4.5083) projected
  arc A91 (22.0512, -4.729) -> (22.3962, -4.7616) centre (22.4322, -2.5424) ccw projected
  arc A92 (22.3962, -4.7616) -> (23.5219, -4.6848) centre (22.545, 1.3418) ccw projected
  arc A93 (23.5219, -4.6848) -> (25.6744, -4.1017) centre (21.852, 5.7456) ccw projected
  arc A94 (25.6744, -4.1017) -> (25.8612, -2.6831) centre (0, 0) ccw projected
  arc A95 (25.8612, -2.6831) -> (23.9329, -1.5628) centre (19.6203, -11.2055) ccw projected
  arc A96 (23.9329, -1.5628) -> (22.8655, -1.1972) centre (21.4295, -7.1312) ccw projected
  arc A97 (22.8655, -1.1972) -> (22.5238, -1.1394) centre (22.3258, -3.3501) ccw projected
  line L24 (21.4725, -1.0863) -> (22.5238, -1.1394) projected
  arc A98 (21.4725, -1.0863) -> (21.4725, 1.0863) centre (0, 0) ccw projected
  line L25 (22.5238, 1.1394) -> (21.4725, 1.0863) projected
  arc A99 (22.5238, 1.1394) -> (22.8655, 1.1972) centre (22.3258, 3.3501) ccw projected
  arc A100 (22.8655, 1.1972) -> (23.9329, 1.5628) centre (21.4295, 7.1312) ccw projected
  arc A101 (23.9329, 1.5628) -> (25.8612, 2.6831) centre (19.6203, 11.2055) ccw projected
  arc A102 (25.8612, 2.6831) -> (25.6744, 4.1017) centre (0, 0) ccw projected
  arc A103 (25.6744, 4.1017) -> (23.5219, 4.6848) centre (21.852, -5.7456) ccw projected
  arc A104 (23.5219, 4.6848) -> (22.3962, 4.7616) centre (22.545, -1.3418) ccw projected
  arc A105 (22.3962, 4.7616) -> (22.0512, 4.729) centre (22.4322, 2.5424) ccw projected
  line L26 (21.022, 4.5083) -> (22.0512, 4.729) projected
  arc A106 (21.022, 4.5083) -> (20.4597, 6.6068) centre (0, 0) ccw projected
  line L27 (21.4614, 6.9302) -> (20.4597, 6.6068) projected
  arc A107 (21.4614, 6.9302) -> (21.7765, 7.0744) centre (20.698, 9.0143) ccw projected
  arc A108 (21.7765, 7.0744) -> (22.713, 7.7038) centre (18.8536, 12.4346) ccw projected
  arc A109 (22.713, 7.7038) -> (24.2856, 9.285) centre (16.0516, 15.9018) ccw projected
  arc A110 (24.2856, 9.285) -> (23.738, 10.607) centre (0, 0) ccw projected
  arc A111 (23.738, 10.607) -> (21.5079, 10.613) centre (22.5945, 0.1059) ccw projected
  arc A112 (21.5079, 10.613) -> (20.4007, 10.3959) centre (22.1241, 4.539) ccw projected
  arc A113 (20.4007, 10.3959) -> (20.0759, 10.2751) centre (21.0098, 8.2616) ccw projected
  line L28 (19.1389, 9.7955) -> (20.0759, 10.2751) projected
  arc A114 (19.1389, 9.7955) -> (18.0526, 11.677) centre (0, 0) ccw projected
  line L29 (18.9365, 12.2487) -> (18.0526, 11.677) projected
  arc A115 (18.9365, 12.2487) -> (19.2035, 12.4696) centre (17.6597, 14.0642) ccw projected
  arc A116 (19.2035, 12.4696) -> (19.9451, 13.3199) centre (14.9929, 16.8905) ccw projected
  arc A117 (19.9451, 13.3199) -> (21.0549, 15.2542) centre (11.389, 19.5144) ccw projected
  arc A118 (21.0549, 15.2542) -> (20.1838, 16.3894) centre (0, 0) ccw projected
  arc A119 (20.1838, 16.3894) -> (18.0282, 15.8181) centre (21.7972, 5.9502) ccw projected
  arc A120 (18.0282, 15.8181) -> (17.0149, 15.3218) centre (20.1955, 10.1104) ccw projected
  arc A121 (17.0149, 15.3218) -> (16.7325, 15.121) centre (18.1556, 13.4178) ccw projected
  line L30 (15.9515, 14.4153) -> (16.7325, 15.121) projected
  arc A122 (15.9515, 14.4153) -> (14.4153, 15.9515) centre (0, 0) ccw projected
  line L31 (15.121, 16.7325) -> (14.4153, 15.9515) projected
  arc A123 (15.121, 16.7325) -> (15.3218, 17.0149) centre (13.4178, 18.1556) ccw projected
  arc A124 (15.3218, 17.0149) -> (15.8181, 18.0282) centre (10.1104, 20.1955) ccw projected
  arc A125 (15.8181, 18.0282) -> (16.3894, 20.1838) centre (5.9502, 21.7972) ccw projected
  arc A126 (16.3894, 20.1838) -> (15.2542, 21.0549) centre (0, 0) ccw projected
  arc A127 (15.2542, 21.0549) -> (13.3199, 19.9451) centre (19.5144, 11.389) ccw projected
  arc A128 (13.3199, 19.9451) -> (12.4696, 19.2035) centre (16.8905, 14.9929) ccw projected
  arc A129 (12.4696, 19.2035) -> (12.2487, 18.9365) centre (14.0642, 17.6597) ccw projected
  line L32 (11.677, 18.0526) -> (12.2487, 18.9365) projected
  arc A130 (11.677, 18.0526) -> (9.7955, 19.1389) centre (0, 0) ccw projected
  line L33 (10.2751, 20.0759) -> (9.7955, 19.1389) projected
  arc A131 (10.2751, 20.0759) -> (10.3959, 20.4007) centre (8.2616, 21.0098) ccw projected
  arc A132 (10.3959, 20.4007) -> (10.613, 21.5079) centre (4.539, 22.1241) ccw projected
  arc A133 (10.613, 21.5079) -> (10.607, 23.738) centre (0.1059, 22.5945) ccw projected
  arc A134 (10.607, 23.738) -> (9.285, 24.2856) centre (0, 0) ccw projected
  arc A135 (9.285, 24.2856) -> (7.7038, 22.713) centre (15.9018, 16.0516) ccw projected
  arc A136 (7.7038, 22.713) -> (7.0744, 21.7765) centre (12.4346, 18.8536) ccw projected
  arc A137 (7.0744, 21.7765) -> (6.9302, 21.4614) centre (9.0143, 20.698) ccw projected
  line L34 (6.6068, 20.4597) -> (6.9302, 21.4614) projected
  arc A138 (6.6068, 20.4597) -> (4.5083, 21.022) centre (0, 0) ccw projected
  line L35 (4.729, 22.0512) -> (4.5083, 21.022) projected
  arc A139 (4.729, 22.0512) -> (4.7616, 22.3962) centre (2.5424, 22.4322) ccw projected
  arc A140 (4.7616, 22.3962) -> (4.6848, 23.5219) centre (-1.3418, 22.545) ccw projected
  arc A141 (4.6848, 23.5219) -> (4.1017, 25.6744) centre (-5.7456, 21.852) ccw projected
  arc A142 (4.1017, 25.6744) -> (2.6831, 25.8612) centre (0, 0) ccw projected
  arc A143 (2.6831, 25.8612) -> (1.5628, 23.9329) centre (11.2055, 19.6203) ccw projected
  arc A144 (1.5628, 23.9329) -> (1.1972, 22.8655) centre (7.1312, 21.4295) ccw projected
  arc A145 (1.1972, 22.8655) -> (1.1394, 22.5238) centre (3.3501, 22.3258) ccw projected
  line L36 (1.0863, 21.4725) -> (1.1394, 22.5238) projected
  arc A146 (1.0863, 21.4725) -> (-1.0863, 21.4725) centre (0, 0) ccw projected
  line L37 (-1.1394, 22.5238) -> (-1.0863, 21.4725) projected
  arc A147 (-1.1394, 22.5238) -> (-1.1972, 22.8655) centre (-3.3501, 22.3258) ccw projected
  arc A148 (-1.1972, 22.8655) -> (-1.5628, 23.9329) centre (-7.1312, 21.4295) ccw projected
  arc A149 (-1.5628, 23.9329) -> (-2.6831, 25.8612) centre (-11.2055, 19.6203) ccw projected
  arc A150 (-2.6831, 25.8612) -> (-4.1017, 25.6744) centre (0, 0) ccw projected
  arc A151 (-4.1017, 25.6744) -> (-4.6848, 23.5219) centre (5.7456, 21.852) ccw projected
  arc A152 (-4.6848, 23.5219) -> (-4.7616, 22.3962) centre (1.3418, 22.545) ccw projected
  arc A153 (-4.7616, 22.3962) -> (-4.729, 22.0512) centre (-2.5424, 22.4322) ccw projected
  line L38 (-4.5083, 21.022) -> (-4.729, 22.0512) projected
  arc A154 (-4.5083, 21.022) -> (-6.6068, 20.4597) centre (0, 0) ccw projected
  line L39 (-6.9302, 21.4614) -> (-6.6068, 20.4597) projected
  arc A155 (-6.9302, 21.4614) -> (-7.0744, 21.7765) centre (-9.0143, 20.698) ccw projected
  arc A156 (-7.0744, 21.7765) -> (-7.7038, 22.713) centre (-12.4346, 18.8536) ccw projected
  arc A157 (-7.7038, 22.713) -> (-9.285, 24.2856) centre (-15.9018, 16.0516) ccw projected
  arc A158 (-9.285, 24.2856) -> (-10.607, 23.738) centre (0, 0) ccw projected
  arc A159 (-10.607, 23.738) -> (-10.613, 21.5079) centre (-0.1059, 22.5945) ccw projected
  arc A160 (-10.613, 21.5079) -> (-10.3959, 20.4007) centre (-4.539, 22.1241) ccw projected
  arc A161 (-10.3959, 20.4007) -> (-10.2751, 20.0759) centre (-8.2616, 21.0098) ccw projected
  line L40 (-9.7955, 19.1389) -> (-10.2751, 20.0759) projected
  arc A162 (-9.7955, 19.1389) -> (-11.677, 18.0526) centre (0, 0) ccw projected
  line L41 (-12.2487, 18.9365) -> (-11.677, 18.0526) projected
  arc A163 (-12.2487, 18.9365) -> (-12.4696, 19.2035) centre (-14.0642, 17.6597) ccw projected
  arc A164 (-12.4696, 19.2035) -> (-13.3199, 19.9451) centre (-16.8905, 14.9929) ccw projected
  arc A165 (-13.3199, 19.9451) -> (-15.2542, 21.0549) centre (-19.5144, 11.389) ccw projected
  arc A166 (-15.2542, 21.0549) -> (-16.3894, 20.1838) centre (0, 0) ccw projected
  arc A167 (-16.3894, 20.1838) -> (-15.8181, 18.0282) centre (-5.9502, 21.7972) ccw projected
  arc A168 (-15.8181, 18.0282) -> (-15.3218, 17.0149) centre (-10.1104, 20.1955) ccw projected
  arc A169 (-15.3218, 17.0149) -> (-15.121, 16.7325) centre (-13.4178, 18.1556) ccw projected
  line L42 (-14.4153, 15.9515) -> (-15.121, 16.7325) projected
  arc A170 (-14.4153, 15.9515) -> (-15.9515, 14.4153) centre (0, 0) ccw projected
  line L43 (-16.7325, 15.121) -> (-15.9515, 14.4153) projected
  arc A171 (-16.7325, 15.121) -> (-17.0149, 15.3218) centre (-18.1556, 13.4178) ccw projected
  arc A172 (-17.0149, 15.3218) -> (-18.0282, 15.8181) centre (-20.1955, 10.1104) ccw projected
  arc A173 (-18.0282, 15.8181) -> (-20.1838, 16.3894) centre (-21.7972, 5.9502) ccw projected
  arc A174 (-20.1838, 16.3894) -> (-21.0549, 15.2542) centre (0, 0) ccw projected
  arc A175 (-21.0549, 15.2542) -> (-19.9451, 13.3199) centre (-11.389, 19.5144) ccw projected
  arc A176 (-19.9451, 13.3199) -> (-19.2035, 12.4696) centre (-14.9929, 16.8905) ccw projected
  arc A177 (-19.2035, 12.4696) -> (-18.9365, 12.2487) centre (-17.6597, 14.0642) ccw projected
  line L44 (-18.0526, 11.677) -> (-18.9365, 12.2487) projected
  arc A178 (-18.0526, 11.677) -> (-19.1389, 9.7955) centre (0, 0) ccw projected
  line L45 (-20.0759, 10.2751) -> (-19.1389, 9.7955) projected
  arc A179 (-20.0759, 10.2751) -> (-20.4007, 10.3959) centre (-21.0098, 8.2616) ccw projected
  arc A180 (-20.4007, 10.3959) -> (-21.5079, 10.613) centre (-22.1241, 4.539) ccw projected
  arc A181 (-21.5079, 10.613) -> (-23.738, 10.607) centre (-22.5945, 0.1059) ccw projected
  arc A182 (-23.738, 10.607) -> (-24.2856, 9.285) centre (0, 0) ccw projected
  arc A183 (-24.2856, 9.285) -> (-22.713, 7.7038) centre (-16.0516, 15.9018) ccw projected
  arc A184 (-22.713, 7.7038) -> (-21.7765, 7.0744) centre (-18.8536, 12.4346) ccw projected
  arc A185 (-21.7765, 7.0744) -> (-21.4614, 6.9302) centre (-20.698, 9.0143) ccw projected
  line L46 (-20.4597, 6.6068) -> (-21.4614, 6.9302) projected
  arc A186 (-20.4597, 6.6068) -> (-21.022, 4.5083) centre (0, 0) ccw projected
  line L47 (-22.0512, 4.729) -> (-21.022, 4.5083) projected
  arc A187 (-22.0512, 4.729) -> (-22.3962, 4.7616) centre (-22.4322, 2.5424) ccw projected
  arc A188 (-22.3962, 4.7616) -> (-23.5219, 4.6848) centre (-22.545, -1.3418) ccw projected
  arc A189 (-23.5219, 4.6848) -> (-25.6744, 4.1017) centre (-21.852, -5.7456) ccw projected
  arc A190 (-25.6744, 4.1017) -> (-25.8612, 2.6831) centre (0, 0) ccw projected
  arc A191 (-25.8612, 2.6831) -> (-23.9329, 1.5628) centre (-19.6203, 11.2055) ccw projected
  arc A192 (-23.9329, 1.5628) -> (-22.8655, 1.1972) centre (-21.4295, 7.1312) ccw projected
  arc A193 (-22.8655, 1.1972) -> (-22.5238, 1.1394) centre (-22.3258, 3.3501) ccw projected
  line L48 (-21.4725, 1.0863) -> (-22.5238, 1.1394) projected
  arc A194 (-21.4725, 1.0863) -> (-21.4725, -1.0863) centre (0, 0) ccw projected
  line L49 (-22.5238, -1.1394) -> (-21.4725, -1.0863) projected
  arc A195 (-22.5238, -1.1394) -> (-22.8655, -1.1972) centre (-22.3258, -3.3501) ccw projected
  arc A196 (-22.8655, -1.1972) -> (-23.9329, -1.5628) centre (-21.4295, -7.1312) ccw projected
  arc A197 (-23.9329, -1.5628) -> (-25.8612, -2.6831) centre (-19.6203, -11.2055) ccw projected
  arc A198 (-25.8612, -2.6831) -> (-25.6744, -4.1017) centre (0, 0) ccw projected
  arc A199 (-25.6744, -4.1017) -> (-23.5219, -4.6848) centre (-21.852, 5.7456) ccw projected
  arc A200 (-23.5219, -4.6848) -> (-22.3962, -4.7616) centre (-22.545, 1.3418) ccw projected
  arc A201 (-22.3962, -4.7616) -> (-22.0512, -4.729) centre (-22.4322, -2.5424) ccw projected
  line L50 (-21.022, -4.5083) -> (-22.0512, -4.729) projected
  arc A202 (-21.022, -4.5083) -> (-20.4597, -6.6068) centre (0, 0) ccw projected
  line L51 (-21.4614, -6.9302) -> (-20.4597, -6.6068) projected
  arc A203 (-21.4614, -6.9302) -> (-21.7765, -7.0744) centre (-20.698, -9.0143) ccw projected
  arc A204 (-21.7765, -7.0744) -> (-22.713, -7.7038) centre (-18.8536, -12.4346) ccw projected
  arc A205 (-22.713, -7.7038) -> (-24.2856, -9.285) centre (-16.0516, -15.9018) ccw projected
  arc A206 (-24.2856, -9.285) -> (-23.738, -10.607) centre (0, 0) ccw projected
  arc A207 (-23.738, -10.607) -> (-21.5079, -10.613) centre (-22.5945, -0.1059) ccw projected
  arc A208 (-21.5079, -10.613) -> (-20.4007, -10.3959) centre (-22.1241, -4.539) ccw projected
  arc A209 (-20.4007, -10.3959) -> (-20.0759, -10.2751) centre (-21.0098, -8.2616) ccw projected
  line L52 (-19.1389, -9.7955) -> (-20.0759, -10.2751) projected
  arc A210 (-19.1389, -9.7955) -> (-18.0526, -11.677) centre (0, 0) ccw projected
  line L53 (-18.9365, -12.2487) -> (-18.0526, -11.677) projected
  arc A211 (-18.9365, -12.2487) -> (-19.2035, -12.4696) centre (-17.6597, -14.0642) ccw projected
  arc A212 (-19.2035, -12.4696) -> (-19.9451, -13.3199) centre (-14.9929, -16.8905) ccw projected
  arc A213 (-19.9451, -13.3199) -> (-21.0549, -15.2542) centre (-11.389, -19.5144) ccw projected
  arc A214 (-21.0549, -15.2542) -> (-20.1838, -16.3894) centre (0, 0) ccw projected
  arc A215 (-20.1838, -16.3894) -> (-18.0282, -15.8181) centre (-21.7972, -5.9502) ccw projected
  arc A216 (-18.0282, -15.8181) -> (-17.0149, -15.3218) centre (-20.1955, -10.1104) ccw projected
  arc A217 (-17.0149, -15.3218) -> (-16.7325, -15.121) centre (-18.1556, -13.4178) ccw projected
  line L54 (-15.9515, -14.4153) -> (-16.7325, -15.121) projected
  arc A218 (-15.9515, -14.4153) -> (-14.4153, -15.9515) centre (0, 0) ccw projected
  line L55 (-15.121, -16.7325) -> (-14.4153, -15.9515) projected
  arc A219 (-15.121, -16.7325) -> (-15.3218, -17.0149) centre (-13.4178, -18.1556) ccw projected
  arc A220 (-15.3218, -17.0149) -> (-15.8181, -18.0282) centre (-10.1104, -20.1955) ccw projected
extrude "押し出し5" add sketch "スケッチ5" against normal blind 0.7 contours A0 A1 L0 A2 A3 A4 L1 A5 | L2 A6 A7 A8 L3 A9 A10 A11 | A13 L4 A14 A15 A16 L5 A17 A12 | A19 L6 A20 A21 A22 L7 A23 A18
equation "\"d13\" = d12"
equation "\"d14\" = d13"
equation "\"d15\" = d14"
equation "\"d16\" = d15"
equation "\"d17\" = d16"
equation "\"d18\" = d13"
equation "\"d19\" = d12"
equation "\"d21\" = d20"
equation "\"d22\" = d21"
equation "\"d23\" = d22"
equation "\"d24\" = d23"
equation "\"d25\" = d23"
equation "\"d26\" = d20"
equation "\"d27\" = d26"
